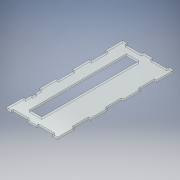
# Autodesk Inventor part: Enclosure Top
Saved by Autodesk Inventor 2018 (Build 220112000, 112)
## iProperties
Created: 2017-12-06
Part Number: Enclosure Top
Material: Glass
Document SubType Name: Modeling
Designer: Andrew
Density: 2.18 g/cm^3
Appearance: Clear
encThick: 0.130 in
encTab: 1.000 in
antOffset: 1.593 in
Author: Andrew
Autodesk Inventor part; units mm, degrees
ref_plane "YZ Plane" through (0, 0, 0) normal (1, 0, 0) x (0, 1, 0)
ref_plane "XZ Plane" through (0, 0, 0) normal (0, 1, 0) x (-1, 0, 0)
ref_plane "XY Plane" through (0, 0, 0) normal (0, 0, 1) x (1, 0, 0)
sketch "Sketch1" plane through (0, 0, 0) normal (0, 1, 0) x (-1, 0, 0)
  line L0 (-38.1, 90.4875) -> (38.1, 90.4875) construction
  line L1 (38.1, 90.4875) -> (38.1, -90.4875) construction
  line L2 (38.1, -90.4875) -> (-38.1, -90.4875) construction
  line L3 (-38.1, -90.4875) -> (-38.1, 90.4875) construction
  line L4 (-38.1, 90.4875) -> (38.1, -90.4875) construction
  line L5 (38.1, 90.4875) -> (-38.1, -90.4875) construction
  line L6 (19.05, 77.7875) -> (0, 77.7875) construction
  line L7 (0, 77.7875) -> (0, -77.7875) construction
  line L8 (0, -77.7875) -> (19.05, -77.7875) construction
  line L9 (19.05, -77.7875) -> (19.05, 77.7875) construction
  line L10 (41.402, 93.7895) -> (-41.402, 93.7895)
  line L11 (-41.402, 93.7895) -> (-41.402, -93.7895)
  line L12 (-41.402, -93.7895) -> (41.402, -93.7895)
  line L13 (41.402, -93.7895) -> (41.402, 93.7895)
  line L14 (41.402, 93.7895) -> (-41.402, -93.7895) construction
  line L15 (-41.402, 93.7895) -> (41.402, -93.7895) construction
  line L16 (19.685, -78.4225) -> (-0.635, -78.4225)
  line L17 (-0.635, -78.4225) -> (-0.635, 78.4225)
  line L18 (-0.635, 78.4225) -> (19.685, 78.4225)
  line L19 (19.685, 78.4225) -> (19.685, -78.4225)
  point P0 (0, 0)
  point P1 (0, 0)
  point P2 (0, 0)
  point P3 (9.525, -78.4225)
  point P4 (9.525, -77.7875)
  point P5 (19.685, 0)
  point P6 (19.05, 0)
  dimension "d0" = 19.05
  dimension "d1" = 155.575
  dimension "d2" = 3.302
  dimension "d3" = 3.302
  dimension "d4" = 12.7
  dimension "d5" = 19.05
  dimension "d6" = 38.1
  dimension "d7" = 0.635
  dimension "d8" = 0.635
  constraints: 40 end point, 10 midpoint, 8 parallel, 4 horizontal, 4 perpendicular, 1 coincident, 1 horizontal alignment, 1 vertical alignment
  measures "d0" distance of L6.start L6.end
  measures "d1" distance of L8.end L6.start
  measures "d2" distance between parallel lines of L12 L2
  measures "d3" distance between parallel lines of L13 L1
  measures "d4" distance between parallel lines of L8 L2
  measures "d5" distance between parallel lines of L1 L9
  measures "d6" distance between parallel lines of L3 L7
  measures "d7" distance between parallel lines of L8 L16
  measures "d8" distance between parallel lines of L9 L19
extrude "Extrusion1" add sketch "Sketch1" along normal blind 3.302
sketch "Sketch2" plane through (0, 0, 0) normal (0, 1, 0) x (-1, 0, 0)
  line L0 (-41.402, 93.7895) -> (-41.402, -93.7895) projected
  line L1 (-41.402, -93.7895) -> (41.402, -93.7895) projected
  line L2 (41.402, -93.7895) -> (41.402, 93.7895) projected
  line L3 (41.402, 93.7895) -> (-41.402, 93.7895) projected
  line L4 (33.576, -93.7895) -> (7.826, -93.7895)
  line L5 (7.826, -93.7895) -> (7.826, -90.4875)
  line L6 (7.826, -90.4875) -> (33.576, -90.4875)
  line L7 (33.576, -90.4875) -> (33.576, -93.7895)
  line L8 (-7.826, -93.7895) -> (-33.576, -93.7895)
  line L9 (-33.576, -93.7895) -> (-33.576, -90.4875)
  line L10 (-33.576, -90.4875) -> (-7.826, -90.4875)
  line L11 (-7.826, -90.4875) -> (-7.826, -93.7895)
  line L12 (0, -131.3053) -> (0, 131.3053) projected
  line L13 (-66.8528, 0) -> (66.8528, 0) projected
  line L14 (-41.402, -66.2073) -> (-38.1, -66.2073)
  line L15 (-38.1, -66.2073) -> (-38.1, -40.4572)
  line L16 (-38.1, -40.4572) -> (-41.402, -40.4572)
  line L17 (-41.402, -40.4572) -> (-41.402, -66.2073)
  line L18 (-41.402, -12.875) -> (-38.1, -12.875)
  line L19 (-38.1, -12.875) -> (-38.1, 12.875)
  line L20 (-38.1, 12.875) -> (-41.402, 12.875)
  line L21 (-41.402, 12.875) -> (-41.402, -12.875)
  line L22 (-41.402, 40.4572) -> (-38.1, 40.4572)
  line L23 (-38.1, 40.4572) -> (-38.1, 66.2073)
  line L24 (-38.1, 66.2073) -> (-41.402, 66.2073)
  line L25 (-41.402, 66.2073) -> (-41.402, 40.4572)
  line L26 (38.1, 50.3478) -> (36.5506, 50.3477)
  line L27 (36.5506, 50.3477) -> (36.5506, 56.3167)
  line L28 (36.5506, 56.3167) -> (38.1, 56.3167)
  line L29 (38.1, 56.3167) -> (38.1, 50.3478)
  point P0 (0, 0)
  point P1 (20.701, -90.4875)
  point P2 (-38.1, -53.3322)
  point P3 (36.5506, 53.3322)
  point P4 (-38.1, 53.3322)
  dimension "d11" = 25.75
  dimension "d13" = 3.302
  dimension "d14" = 41.402
  dimension "d15" = 20.701
  dimension "d19" = 3.302
  dimension "d24" = 40.4573
  dimension "d25" = 80.9145
  dimension "d33" = 1.5494
  dimension "d34" = 5.969
  dimension "d35" = 3.302
  dimension "d36" = 40.4573
  constraints: 48 end point, 12 parallel, 8 point on line, 6 horizontal, 6 perpendicular, 4 equal length, 4 midpoint, 1 horizontal alignment, 3 other
  measures "d11" distance of L5.end L6.end
  measures "d13" distance of L6.end L4.start
  measures "d14" distance between parallel lines of L2 L12
  measures "d15" distance from line of L12 point (20.701, -90.487)
  measures "d19" distance of L14.start L14.end
  measures "d24" distance from line of point (-38.1, -53.332) L1
  measures "d25" distance between parallel lines of L18 L1
  measures "d33" distance of L26.start L26.end
  measures "d34" distance of L26.end L27.end
  measures "d35" distance between parallel lines of L2 L29
  measures "d36" distance from line of L3 point (36.551, 53.332)
extrude "Extrusion2" cut sketch "Sketch2" along normal blind 3.302 contours L24 L23 L22 L0 | L20 L19 L13 L0 | L19 L18 L0 L13 | L16 L15 L14 L0
extrude "Extrusion3" cut sketch "Sketch2" along normal blind 3.302 contours L1 L9 L10 L11 | L5 L6 L7 L1
mirror "Mirror1" about plane through (0, 0, 0) normal (1, 0, 0) of "Extrusion2"
mirror "Mirror2" about plane through (0, 0, 0) normal (0, 0, 1) of "Extrusion3"
extrude "Extrusion4" cut sketch "Sketch2" along normal blind 3.302 contours L26 L27 L28 L29
equation "\"d2\" = encThick"
equation "\"d3\" = encThick"
equation "\"d9\" = encThick"
equation "\"d13\" = encThick"
equation "\"d15\" = 0.5 * d14"
equation "\"d19\" = d13"
equation "\"d24\" = 0.5 * d25"
equation "\"d35\" = encThick"
equation "\"d26\" = encThick"
equation "\"d28\" = encThick"
equation "\"d37\" = encThick"
equation "\"encThick\" = 3.302"
equation "\"encTab\" = 25.4"
equation "\"antOffset\" = d36"
body "Solid1"
